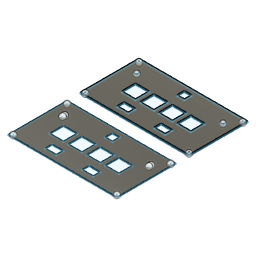
사볼콘 v5 (Autodesk Fusion 360 design; units mm, degrees)
Autodesk Fusion 360 part; units mm, degrees
sketch "스케치1" plane through (0, 0, 0) normal (0, 0, 1) x (1, 0, 0)
  line L0 (-63, 91.5) -> (389, 91.5)
  line L1 (389, 91.5) -> (389, -152.5)
  line L2 (389, -152.5) -> (-63, -152.5)
  line L3 (-63, -152.5) -> (-63, 91.5)
  circle A0 centre (-17, 35.5) radius 4.65
  circle A1 centre (-17, 26.5) radius 1.65
  circle A2 centre (343, 35.5) radius 4.65
  circle A3 centre (343, 26.5) radius 1.65
  line L4 (148, 69.5) -> (178, 69.5)
  line L5 (178, 69.5) -> (178, 39.5)
  line L6 (178, 39.5) -> (148, 39.5)
  line L7 (148, 39.5) -> (148, 69.5)
  line L8 (19, -5.5) -> (76, -5.5)
  line L9 (76, -5.5) -> (76, -62.5)
  line L10 (76, -62.5) -> (19, -62.5)
  line L11 (19, -62.5) -> (19, -5.5)
  line L12 (96, -5.5) -> (153, -5.5)
  line L13 (153, -5.5) -> (153, -62.5)
  line L14 (153, -62.5) -> (96, -62.5)
  line L15 (96, -62.5) -> (96, -5.5)
  line L16 (173, -5.5) -> (230, -5.5)
  line L17 (230, -5.5) -> (230, -62.5)
  line L18 (230, -62.5) -> (173, -62.5)
  line L19 (173, -62.5) -> (173, -5.5)
  line L20 (250, -5.5) -> (307, -5.5)
  line L21 (307, -5.5) -> (307, -62.5)
  line L22 (307, -62.5) -> (250, -62.5)
  line L23 (250, -62.5) -> (250, -5.5)
  line L24 (63, -96.5) -> (109, -96.5)
  line L25 (109, -96.5) -> (109, -125.5)
  line L26 (109, -125.5) -> (63, -125.5)
  line L27 (63, -125.5) -> (63, -96.5)
  line L28 (217, -96.5) -> (263, -96.5)
  line L29 (263, -96.5) -> (263, -125.5)
  line L30 (263, -125.5) -> (217, -125.5)
  line L31 (217, -125.5) -> (217, -96.5)
  circle A4 centre (-53, -142.5) radius 2
  circle A5 centre (-53, 81.5) radius 2
  circle A6 centre (379, 81.5) radius 2
  circle A7 centre (379, -142.5) radius 2
  dimension "d1" = 452
  dimension "d2" = 244
  dimension "d3" = 9.3
  dimension "d4" = 46
  dimension "d5" = 56
  dimension "d6" = 3.3
  dimension "d7" = 9
  dimension "d8" = 9.3
  dimension "d9" = 46
  dimension "d10" = 56
  dimension "d11" = 3.3
  dimension "d12" = 9
  dimension "d13" = 30
  dimension "d14" = 30
  dimension "d15" = 22
  dimension "d16" = 211
  dimension "d17" = 57
  dimension "d18" = 57
  dimension "d19" = 82
  dimension "d20" = 97
  dimension "d21" = 57
  dimension "d22" = 57
  dimension "d23" = 20
  dimension "d24" = 57
  dimension "d25" = 57
  dimension "d26" = 20
  dimension "d27" = 57
  dimension "d28" = 57
  dimension "d29" = 20
  dimension "d124" = 46
  dimension "d125" = 29
  dimension "d126" = 126
  dimension "d127" = 27
  dimension "d128" = 46
  dimension "d129" = 29
  dimension "d130" = 108
  dimension "d131" = 4
  dimension "d132" = 10
  dimension "d133" = 10
  dimension "d134" = 4
  dimension "d135" = 10
  dimension "d136" = 10
  dimension "d137" = 4
  dimension "d138" = 10
  dimension "d139" = 10
  dimension "d140" = 4
  dimension "d141" = 10
  dimension "d142" = 10
  constraint horizontal L0
  constraint vertical L1
  constraint horizontal L2
  constraint vertical L3
  constraint vertical A0.centre A1.centre
  constraint vertical A2.centre A3.centre
  constraint horizontal L4
  constraint vertical L5
  constraint horizontal L6
  constraint vertical L7
  constraint horizontal L8
  constraint vertical L9
  constraint horizontal L10
  constraint vertical L11
  constraint horizontal L12
  constraint vertical L13
  constraint horizontal L14
  constraint vertical L15
  constraint collinear L8 L12
  constraint horizontal L16
  constraint vertical L17
  constraint horizontal L18
  constraint vertical L19
  constraint collinear L12 L16
  constraint horizontal L20
  constraint vertical L21
  constraint horizontal L22
  constraint vertical L23
  constraint collinear L16 L20
  constraint horizontal L24
  constraint vertical L25
  constraint horizontal L26
  constraint vertical L27
  constraint horizontal L28
  constraint vertical L29
  constraint horizontal L30
  constraint vertical L31
  constraint collinear L24 L28
  measures "d1" distance of L0.start L0.end
  measures "d2" distance of L0.start L2.end
  measures "d3" diameter of A0
  measures "d4" distance of L3 A0.centre
  measures "d5" distance of L0 A0.centre
  measures "d6" diameter of A1
  measures "d7" distance of A0.centre A1.centre
  measures "d8" diameter of A2
  measures "d9" distance of L1 A2.centre
  measures "d10" distance of L0 A2.centre
  measures "d11" diameter of A3
  measures "d12" distance of A2.centre A3.centre
  measures "d13" distance of L4.start L4.end
  measures "d14" distance of L4.start L6.end
  measures "d15" distance of L0 L4
  measures "d16" distance of L3 L7
  measures "d17" distance of L8.start L8.end
  measures "d18" distance of L8.start L10.end
  measures "d19" distance of L3 L11
  measures "d20" distance of L0 L8
  measures "d21" distance of L12.start L12.end
  measures "d22" distance of L12.start L14.end
  measures "d23" distance of L9 L15
  measures "d24" distance of L16.start L16.end
  measures "d25" distance of L16.start L18.end
  measures "d26" distance of L13 L19
  measures "d27" distance of L20.start L20.end
  measures "d28" distance of L20.start L22.end
  measures "d29" distance of L17 L23
  measures "d124" distance of L24.start L24.end
  measures "d125" distance of L24.start L26.end
  measures "d126" distance of L3 L27
  measures "d127" distance of L2 L26
  measures "d128" distance of L28.start L28.end
  measures "d129" distance of L28.start L30.end
  measures "d130" distance of L25 L31
  measures "d131" diameter of A4
  measures "d132" distance of L3 A4.centre
  measures "d133" distance of L2 A4.centre
  measures "d134" diameter of A5
  measures "d135" distance of L0 A5.centre
  measures "d136" distance of L3 A5.centre
  measures "d137" diameter of A6
  measures "d138" distance of L0 A6.centre
  measures "d139" distance of L1 A6.centre
  measures "d140" diameter of A7
  measures "d141" distance of L1 A7.centre
  measures "d142" distance of L2 A7.centre
sketch "스케치2" plane through (0, 0, 0) normal (0, 0, 1) x (1, 0, 0)
  line L0 (250, 237.5) -> (250, 294.5)
  line L1 (230, 294.5) -> (230, 237.5)
  circle A0 centre (343, 335.5) radius 7.5
  line L2 (173, 294.5) -> (230, 294.5)
  line L3 (153, 237.5) -> (96, 237.5)
  line L4 (19, 237.5) -> (19, 294.5)
  line L5 (-63, 391.5) -> (389, 391.5)
  circle A1 centre (-17, 335.5) radius 7.5
  line L6 (96, 294.5) -> (153, 294.5)
  line L7 (-63, 147.5) -> (-63, 391.5)
  line L8 (19, 294.5) -> (76, 294.5)
  line L9 (178, 339.5) -> (148, 339.5)
  line L10 (148, 369.5) -> (178, 369.5)
  line L11 (307, 237.5) -> (250, 237.5)
  line L12 (178, 369.5) -> (178, 339.5)
  line L13 (389, 391.5) -> (389, 147.5)
  line L14 (173, 237.5) -> (173, 294.5)
  line L15 (76, 237.5) -> (19, 237.5)
  line L16 (230, 237.5) -> (173, 237.5)
  line L17 (153, 294.5) -> (153, 237.5)
  line L18 (96, 237.5) -> (96, 294.5)
  line L19 (76, 294.5) -> (76, 237.5)
  line L20 (250, 294.5) -> (307, 294.5)
  line L21 (389, 147.5) -> (-63, 147.5)
  line L22 (307, 294.5) -> (307, 237.5)
  line L23 (148, 339.5) -> (148, 369.5)
  line L24 (63, 203.5) -> (109, 203.5)
  line L25 (109, 203.5) -> (109, 174.5)
  line L26 (109, 174.5) -> (63, 174.5)
  line L27 (63, 174.5) -> (63, 203.5)
  line L28 (217, 203.5) -> (263, 203.5)
  line L29 (263, 203.5) -> (263, 174.5)
  line L30 (263, 174.5) -> (217, 174.5)
  line L31 (217, 174.5) -> (217, 203.5)
  circle A2 centre (-53, 381.5) radius 2
  circle A3 centre (-53, 157.5) radius 2
  circle A4 centre (379, 381.5) radius 2
  circle A5 centre (379, 157.5) radius 2
  dimension "d47" = 452
  dimension "d48" = 244
  dimension "d49" = 15
  dimension "d50" = 46
  dimension "d51" = 56
  dimension "d54" = 15
  dimension "d55" = 46
  dimension "d56" = 56
  dimension "d59" = 30
  dimension "d60" = 30
  dimension "d61" = 22
  dimension "d62" = 211
  dimension "d63" = 57
  dimension "d64" = 57
  dimension "d65" = 82
  dimension "d66" = 97
  dimension "d67" = 57
  dimension "d68" = 57
  dimension "d69" = 20
  dimension "d70" = 57
  dimension "d71" = 57
  dimension "d72" = 20
  dimension "d73" = 57
  dimension "d74" = 57
  dimension "d75" = 20
  dimension "d117" = 46
  dimension "d118" = 29
  dimension "d119" = 126
  dimension "d120" = 27
  dimension "d121" = 46
  dimension "d122" = 29
  dimension "d123" = 108
  dimension "d179" = 4
  dimension "d180" = 10
  dimension "d181" = 10
  dimension "d182" = 4
  dimension "d183" = 4
  dimension "d184" = 4
  dimension "d185" = 10
  dimension "d186" = 10
  dimension "d187" = 10
  dimension "d188" = 10
  dimension "d189" = 10
  dimension "d190" = 10
  constraint horizontal L5
  constraint vertical L13
  constraint horizontal L21
  constraint vertical L7
  constraint horizontal L10
  constraint vertical L12
  constraint horizontal L9
  constraint vertical L23
  constraint horizontal L8
  constraint vertical L19
  constraint horizontal L15
  constraint vertical L4
  constraint horizontal L6
  constraint vertical L17
  constraint horizontal L3
  constraint vertical L18
  constraint collinear L6 L8
  constraint horizontal L2
  constraint vertical L1
  constraint horizontal L16
  constraint vertical L14
  constraint collinear L2 L6
  constraint horizontal L20
  constraint vertical L22
  constraint horizontal L11
  constraint vertical L0
  constraint collinear L2 L20
  constraint horizontal L24
  constraint vertical L25
  constraint horizontal L26
  constraint vertical L27
  constraint horizontal L28
  constraint vertical L29
  constraint horizontal L30
  constraint vertical L31
  constraint collinear L24 L28
  measures "d47" distance of L5.start L5.end
  measures "d48" distance of L5.start L7.start
  measures "d49" diameter of A1
  measures "d50" distance of A1.centre L7
  measures "d51" distance of A1.centre L5
  measures "d54" diameter of A0
  measures "d55" distance of A0.centre L13
  measures "d56" distance of A0.centre L5
  measures "d59" distance of L10.start L10.end
  measures "d60" distance of L10.start L9.end
  measures "d61" distance of L5 L10
  measures "d62" distance of L7 L23
  measures "d63" distance of L8.end L4.end
  measures "d64" distance of L4.start L4.end
  measures "d65" distance of L4 L7
  measures "d66" distance of L5 L8
  measures "d67" distance of L6.start L6.end
  measures "d68" distance of L6.start L3.end
  measures "d69" distance of L18 L19
  measures "d70" distance of L2.start L1.start
  measures "d71" distance of L2.start L14.start
  measures "d72" distance of L14 L17
  measures "d73" distance of L0.end L20.end
  measures "d74" distance of L0.end L0.start
  measures "d75" distance of L0 L1
  measures "d117" distance of L24.start L24.end
  measures "d118" distance of L24.start L26.end
  measures "d119" distance of L7 L27
  measures "d120" distance of L21 L26
  measures "d121" distance of L28.start L28.end
  measures "d122" distance of L28.start L30.end
  measures "d123" distance of L25 L31
  measures "d179" diameter of A2
  measures "d180" distance of L5 A2.centre
  measures "d181" distance of L7 A2.centre
  measures "d182" diameter of A3
  measures "d183" diameter of A4
  measures "d184" diameter of A5
  measures "d185" distance of L7 A3.centre
  measures "d186" distance of L21 A3.centre
  measures "d187" distance of L5 A4.centre
  measures "d188" distance of L13 A4.centre
  measures "d189" distance of L21 A5.centre
  measures "d190" distance of L13 A5.centre
extrude "돌출4" add sketch "스케치1" along normal blind 2 makes body 1
extrude "돌출7" add sketch "스케치2" along normal blind 5 separate body makes body 2
extrude "돌출2" [suppressed]
hole "홀1" [suppressed]
hole "홀2" [suppressed]
move_body "이동2" [suppressed]
move_body "이동3" [suppressed]
move_body "이동4" [suppressed]
move_body "이동5" [suppressed]
move_body "이동6" [suppressed]
move_body "이동7" [suppressed]
move_body "이동8" [suppressed]
named bodies: "하판", "상판"
